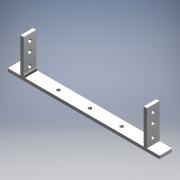
# Autodesk Inventor part: Back Brace
Saved by Autodesk Inventor 2019.4 (Build 234330000, 330)
## iProperties
Created: 2020-01-21
Part Number: Back Brace
Material: Aluminum 6061
Document SubType Name: Modeling
Designer: Mark
Mass: 29.7 g
Surface Area: 57 cm^2
Volume: 11 cm^3
Density: 2.7 g/cm^3
Appearance: Aluminum - Flat
Author: Mark
Autodesk Inventor part; units mm, degrees
ref_plane "YZ Plane" through (0, 0, 0) normal (1, 0, 0) x (0, 1, 0)
ref_plane "XZ Plane" through (0, 0, 0) normal (0, 1, 0) x (-1, 0, 0)
ref_plane "XY Plane" through (0, 0, 0) normal (0, 0, 1) x (1, 0, 0)
sketch "Sketch1" plane through (0, 0, 0) normal (0, 0, 1) x (1, 0, 0)
  line L0 (0, 0) -> (20, 0)
  line L1 (20, 0) -> (20, 5)
  line L2 (20, 5) -> (0, 5)
  line L3 (0, 5) -> (0, 0)
  line L4 (20, 0) -> (25, 0)
  line L5 (25, 0) -> (25, 60)
  line L6 (25, 60) -> (20, 60)
  line L7 (20, 60) -> (20, 0)
  line L8 (25, 0) -> (120, 0)
  line L9 (120, 0) -> (120, 5)
  line L10 (120, 5) -> (25, 5)
  line L11 (25, 5) -> (25, 0)
  line L12 (240, 0) -> (220, 0)
  line L13 (220, 0) -> (220, 5)
  line L14 (220, 5) -> (240, 5)
  line L15 (240, 5) -> (240, 0)
  line L16 (220, 0) -> (215, 0)
  line L17 (215, 0) -> (215, 60)
  line L18 (215, 60) -> (220, 60)
  line L19 (220, 60) -> (220, 0)
  line L20 (215, 0) -> (120, 0)
  line L21 (120, 5) -> (215, 5)
  line L22 (215, 5) -> (215, 0)
  dimension "d0" = 20
  dimension "d1" = 5
  dimension "d2" = 5
  dimension "d3" = 60
  dimension "d4" = 95
  dimension "d5" = 5
  constraints: 46 end point, 8 symmetric about line, 6 parallel, 3 horizontal, 3 perpendicular
  measures "d0" distance of L2.end L1.end
  measures "d1" distance of L1.end L0.end
  measures "d2" distance of L6.end L5.end
  measures "d3" distance of L5.end L4.end
  measures "d4" distance of L10.end L9.end
  measures "d5" distance of L9.end L8.end
extrude "Extrusion1" add sketch "Sketch1" along normal blind 20
fillet "Fillet1" radius 5 1 edges at (25, 5, 10)
sketch "Sketch2" plane through (120, 5, 20) normal (0, 1, 0) x (1, 0, 0)
  circle A0 centre (-50, 10) radius 2.75
  line L0 (95, 0) -> (-90, 0) projected
  line L1 (0, 21.3333) -> (0, 1.3333)
  line L2 (-90, 0) -> (-90, 20) projected
  circle A1 centre (0, 10) radius 2.75
  circle A2 centre (50, 10) radius 2.75
  point P0 (-120, 20)
  dimension "d9" = 5.5
  dimension "d12" = 10
  dimension "d13" = 50
  dimension "d14" = 5.5
  dimension "d15" = 10
  dimension "d16" = 5.5
  dimension "d17" = 50
  dimension "d18" = 10
  dimension "d19" = 90
  constraints: 3 centre point, 2 end point, 1 parallel, 1 point on line
  measures "d9" diameter of A0
  measures "d12" distance from line of L0 A0.centre
  measures "d13" distance from line of L1 A0.centre
  measures "d14" diameter of A1
  measures "d15" distance from line of L0 A1.centre
  measures "d16" diameter of A2
  measures "d17" distance of A1.centre A2.centre
  measures "d18" distance from line of L0 A2.centre
  measures "d19" distance between parallel lines of L2 L1
extrude "Extrusion2" cut sketch "Sketch2" against normal blind 5
sketch "Sketch3" plane through (25, 60, 20) normal (1, 0, 0) x (0, 0, -1)
  circle A0 centre (10, -45) radius 2.75
  circle A1 centre (10, -25) radius 2.75
  line L0 (0, -55) -> (0, 0) projected
  line L1 (20, -55) -> (0, -55) projected
  circle A2 centre (10, -10) radius 2.75
  point P0 (20, -60)
  dimension "d20" = 5.5
  dimension "d21" = 5.5
  dimension "d22" = 10
  dimension "d23" = 10
  dimension "d24" = 20
  dimension "d25" = 10
  dimension "d26" = 5.5
  dimension "d27" = 10
  dimension "d28" = 15
  constraints: 3 centre point
  measures "d20" diameter of A0
  measures "d21" diameter of A1
  measures "d22" distance from line of L0 A1.centre
  measures "d23" distance from line of L0 A0.centre
  measures "d24" distance of A1.centre A0.centre
  measures "d25" distance from line of L1 A0.centre
  measures "d26" diameter of A2
  measures "d27" distance from line of L0 A2.centre
  measures "d28" distance of A1.centre A2.centre
extrude "Extrusion3" cut sketch "Sketch3" along normal through all both and the other way through all
body "Solid1"
